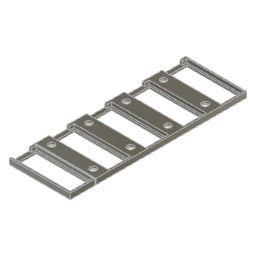
OLED Support for UFC v1 (Autodesk Fusion 360 design; units mm, degrees)
Autodesk Fusion 360 part; units mm, degrees
note: some values were not read from the file. Set by a fixed rule: which face or edge a step refers to.
sketch "Sketch1" plane through (0, 0, 0) normal (0, 0, 1) x (1, 0, 0)
  line L0 (15.1, -5.85) -> (-15.1, -5.85)
  line L1 (-15.1, -5.85) -> (-15.1, 5.85)
  line L2 (-15.1, 5.85) -> (15.1, 5.85)
  line L3 (15.1, 5.85) -> (15.1, -5.85)
  line L4 (15.1, -5.85) -> (-15.1, 5.85) construction
  line L5 (-15.1, -5.85) -> (15.1, 5.85) construction
  line L6 (14.85, -5.4) -> (-14.85, -5.4)
  line L7 (-14.85, -5.4) -> (-14.85, 5.4)
  line L8 (-14.85, 5.4) -> (14.85, 5.4)
  line L9 (14.85, 5.4) -> (14.85, -5.4)
  line L10 (14.85, -5.4) -> (-14.85, 5.4) construction
  line L11 (-14.85, -5.4) -> (14.85, 5.4) construction
  line L12 (16, -7) -> (-16, -7)
  line L13 (-16, -7) -> (-16, 7)
  line L14 (-16, 7) -> (16, 7)
  line L15 (16, 7) -> (16, -7)
  line L16 (16, -7) -> (-16, 7) construction
  line L17 (-16, -7) -> (16, 7) construction
  line L18 (-16, 7) -> (-14.85, 7)
  line L19 (-14.85, 7) -> (-14.85, -3.1641)
  line L20 (-14.85, -3.1641) -> (-16, -3.1641)
  line L21 (-16, -3.1641) -> (-16, 7)
  dimension "d3" = 30.2
  dimension "d4" = 11.7
  dimension "d5" = 29.7
  dimension "d6" = 10.8
  constraint horizontal L0
  constraint perpendicular L0 L1
  constraint parallel L0 L2
  constraint parallel L1 L3
  constraint coincident L4 origin
  constraint coincident L5 origin
  constraint horizontal L6
  constraint perpendicular L6 L7
  constraint parallel L6 L8
  constraint parallel L7 L9
  constraint coincident L10 origin
  constraint coincident L11 origin
  constraint horizontal L12
  constraint perpendicular L12 L13
  constraint parallel L12 L14
  constraint parallel L13 L15
  constraint coincident L16 origin
  constraint coincident L17 origin
  constraint horizontal L18
  constraint vertical L19
  constraint horizontal L20
  constraint vertical L21
  constraint coincident L7 L19.end
  measures "d3" distance of L1.end L2.end
  measures "d4" distance of L0.end L1.end
  measures "d5" distance of L7.end L8.end
  measures "d6" distance of L6.end L7.end
extrude "Extrude1" add sketch "Sketch1" along normal blind 1 contours L0 L1 L2 L3 L6 L7 L8 L9 L19 L20 | L1 L2 L7 L19 L20 makes body 1
extrude "Extrude2" add sketch "Sketch1" along normal blind 4 contours L0 L1 L2 L3 L12 L13 L14 L15 L19 L20 | L1 L2 L13 L14 L18 L19 L20 L21 bodies 1
sketch "Sketch2" plane through (0, 0, 4) normal (0, 0, 1) x (-1, 0, 0)
  line L0 (15.1, -5.85) -> (-15.1, -5.85)
  line L1 (-15.1, -5.85) -> (-15.1, 5.85)
  line L2 (-15.1, 5.85) -> (15.1, 5.85)
  line L3 (15.1, 5.85) -> (15.1, -5.85)
  line L4 (-16, -7) -> (16, -7)
  line L5 (16, -7) -> (16, 7)
  line L6 (16, 7) -> (-16, 7)
  line L7 (-16, 7) -> (-16, -7)
  line L8 (16, 6) -> (15.1, 6)
  line L9 (15.1, 6) -> (15.1, -7)
  line L10 (15.1, -7) -> (16, -7)
  line L11 (16, -7) -> (16, 6)
  constraint horizontal L8
  constraint vertical L9
  constraint horizontal L10
  constraint vertical L11
  constraint coincident L4 L9.end
  constraint coincident L5 L8.start
extrude "Extrude3" cut sketch "Sketch2" against normal blind 4 contours L3 L4 L5 L8 L9 L10 L11 bodies 1
sketch "Sketch3" plane through (-15.1, 0, 0) normal (-1, 0, 0) x (0, -1, 0)
  line L0 (5.85, 1) -> (-5.85, 1)
  line L1 (-5.85, 1) -> (-5.85, 4)
  line L2 (-5.85, 4) -> (-7, 4)
  line L3 (-7, 4) -> (-7, 0)
  line L4 (-7, 0) -> (6, 0)
  line L5 (6, 0) -> (6, 4)
  line L6 (5.85, 4) -> (5.85, 1)
  line L7 (6, 4) -> (5.85, 4)
extrude "Extrude4" add sketch "Sketch3" along normal blind 1 bodies 1
sketch "Sketch4" plane through (0, 5.85, 0) normal (0, -1, 0) x (1, 0, 0)
  line L0 (-16.1, 1) -> (15.1, 1)
  line L1 (15.1, 1) -> (15.1, 4)
  line L2 (15.1, 4) -> (-16.1, 4)
  line L3 (-16.1, 4) -> (-16.1, 1)
  line L4 (-14.8297, 1) -> (-16.1, 1)
  line L5 (-16.1, 1) -> (-16.1, 4)
  line L6 (-16.1, 4) -> (-14.8297, 4)
  line L7 (-14.8297, 4) -> (-14.8297, 1)
  constraint horizontal L4
  constraint vertical L5
  constraint horizontal L6
  constraint vertical L7
  constraint coincident L2.end L3.start
  constraint coincident L0 L4.start
extrude "Extrude5" add sketch "Sketch4" along normal blind 2 contours L0 L2 L3 L4 L5 L6 L7 bodies 1
move_face "OffsetFaces1" offset 1 2 faces at (-16.1, 5.95, 1.6667) (-16, -6.6667, 1.3333) on bodies 1
extrude "Extrude6" cut 1 faces at (-14.8297, 5.0333, 3) along direction (-1, 0, 0) blind 1 on bodies 1 bodies 1
sketch "Sketch5" plane through (0, 0, 0) normal (0, 0, 1) x (1, 0, 0)
  line L0 (15, -6) -> (-15, -6)
  line L1 (-15, -6) -> (-15, 14)
  line L2 (15, 14) -> (15, -6)
  line L3 (15, 54) -> (15, 74)
  line L4 (15, 74) -> (-15, 74)
  line L5 (-15, 74) -> (-15, 54)
  line L6 (-15, -6) -> (15, -6)
  line L7 (15, -6) -> (15, 14.5)
  line L8 (15, 14.5) -> (-15, 14.5)
  line L9 (-15, 14.5) -> (-15, -6)
  line L10 (-15, 14.5) -> (15, 14.5)
  line L11 (15, 14.5) -> (15, 35)
  line L12 (15, 35) -> (-15, 35)
  line L13 (-15, 35) -> (-15, 14.5)
  line L14 (15, 35) -> (15, 55.5)
  line L15 (15, 55.5) -> (-15, 55.5)
  line L16 (-15, 55.5) -> (-15, 35)
  line L17 (-15, 55.5) -> (15, 55.5)
  line L18 (15, 55.5) -> (15, 76)
  line L19 (15, 76) -> (-15, 76)
  line L20 (-15, 76) -> (-15, 55.5)
  dimension "d30" = 30
  dimension "d31" = 20.5
  dimension "d32" = 30
  dimension "d33" = 20.5
  dimension "d34" = 30
  dimension "d35" = 20.5
  dimension "d36" = 30
  dimension "d37" = 20.5
  constraint horizontal L0
  constraint vertical L1
  constraint vertical L2
  constraint vertical L3
  constraint horizontal L4
  constraint vertical L5
  constraint horizontal L6
  constraint vertical L7
  constraint horizontal L8
  constraint vertical L9
  constraint horizontal L10
  constraint vertical L11
  constraint horizontal L12
  constraint vertical L13
  constraint vertical L14
  constraint horizontal L15
  constraint vertical L16
  constraint horizontal L17
  constraint vertical L18
  constraint horizontal L19
  constraint vertical L20
  measures "d30" distance of L0.end L0.start
  measures "d31" distance of L0.end L8.end
  measures "d32" distance of L8.end L7.end
  measures "d33" distance of L8.end L12.end
  measures "d34" distance of L12.end L11.end
  measures "d35" distance of L12.end L15.end
  measures "d36" distance of L15.end L14.end
  measures "d37" distance of L15.end L19.end
copy_body "Body->Comp2" bodies 1 removing the originals makes body 2 in component "Component'"
copy_body "CopyPasteBodies5" bodies 2 makes body 3
move_body "Move5" bodies 3 to x (1, 0, 0) y (0, 1, 0) z (0, 0, 1) at (0, 20.5, 0)
copy_body "CopyPasteBodies6" bodies 3 makes body 4
move_body "Move6" bodies 4 to x (1, 0, 0) y (0, 1, 0) z (0, 0, 1) at (0, 20.5, 0)
copy_body "CopyPasteBodies7" bodies 4 makes body 5
move_body "Move7" bodies 5 to x (1, 0, 0) y (0, 1, 0) z (0, 0, 1) at (0, 20.5, 0)
copy_body "CopyPasteBodies8" bodies 5 makes body 6
move_body "Move8" bodies 6 to x (1, 0, 0) y (0, 1, 0) z (0, 0, 1) at (0, 20.5, 0)
extrude "Extrude12" add 1 faces at (5, 75, 2.6667) along direction (0, -1, 0) blind 7 on bodies 6 bodies 6 5
extrude "Extrude13" add 1 faces at (5, 54.5, 2.6667) along direction (0, -1, 0) blind 8 on bodies 6 bodies 6 4
extrude "Extrude14" add 1 faces at (5, 34, 2.6667) along direction (0, -1, 0) blind 7 on bodies 6 bodies 6 3
extrude "Extrude15" add 1 faces at (5, 13.5, 2.6667) along direction (0, -1, 0) blind 7 on bodies 6 bodies 6
extrude "Extrude16" cut 1 faces at (4.7901, 46.5, 3) along direction (0, 1, 0) blind 0.4 on bodies 6 bodies 6
sketch "Sketch6" plane through (0, 0, 0) normal (0, 0, 1) x (1, 0, 0)
  arc A0 through (-26.4037, -5.2537, 2.667) (-26.7629, -5.1049, 2.667) (-26.9117, -4.7457, 2.667)
  arc A1 through (15.7603, 87.9325, 2.667) (16.1195, 87.7838, 2.667) (16.2683, 87.4245, 2.667)
  circle A2 through (-20.4791, 31.1794, 0.9906) (-22.508, 32.3508, 0.9906) (-22.508, 30.0081, 0.9906)
  arc A3 through (18.3003, -13.0166, 2.667) (18.6595, -12.8678, 2.667) (18.8083, -12.5086, 2.667)
  arc A4 through (-26.4037, 55.7063, 2.667) (-26.7629, 55.8551, 2.667) (-26.9117, 56.2143, 2.667)
  line L0 (13.5696, 95.6954, 0.9906) -> (8.8071, 95.6954, 0.9906)
  line L1 (13.5696, 95.6954, 2.667) -> (18.3003, 95.6954, 2.667)
  arc A5 through (-26.9117, 6.1445, 2.667) (-26.7629, 6.5038, 2.667) (-26.4037, 6.6525, 2.667)
  line L2 (8.8071, 95.6954, 2.667) -> (8.8071, 93.3078, 2.667)
  line L3 (18.8083, 95.1874, 2.667) -> (18.8083, -12.5086, 2.667)
  arc A6 through (8.8071, -10.629, 2.667) (11.1883, -8.2477, 2.667) (13.5696, -10.629, 2.667)
  arc A7 through (15.7603, 67.6125, 2.667) (16.1195, 67.4638, 2.667) (16.2683, 67.1045, 2.667)
  line L4 (-24.2129, -10.629, 2.667) -> (-24.2129, -13.0166, 2.667)
  curve E0
  curve E1
  arc A8 through (-26.9117, 87.4245, 2.667) (-26.7629, 87.7838, 2.667) (-26.4037, 87.9325, 2.667)
  arc A9 through (16.2683, 76.5343, 2.667) (16.1195, 76.1751, 2.667) (15.7603, 76.0263, 2.667)
  circle A10 through (-20.4791, 71.8194, 0.9906) (-22.508, 72.9908, 0.9906) (-22.508, 70.6481, 0.9906)
  arc A11 through (-26.4037, 35.3863, 2.667) (-26.7629, 35.5351, 2.667) (-26.9117, 35.8943, 2.667)
  arc A12 through (-26.9117, 46.7845, 2.667) (-26.7629, 47.1438, 2.667) (-26.4037, 47.2925, 2.667)
  circle A13 through (-20.4791, 93.3078, 0.9906) (-22.508, 94.4792, 0.9906) (-22.508, 92.1365, 0.9906)
  arc A14 through (16.2683, 15.5743, 2.667) (16.1195, 15.2151, 2.667) (15.7603, 15.0663, 2.667)
  line L5 (-26.4037, 76.0263, 2.667) -> (15.7603, 76.0263, 2.667)
  line L6 (-26.4037, 35.3863, 2.667) -> (15.7603, 35.3863, 2.667)
  circle A15 through (12.5409, 51.4994, 0.9906) (10.512, 52.6708, 0.9906) (10.512, 50.3281, 0.9906)
  circle A16 through (8.8071, 10.8594, 2.667) (12.3789, 12.9216, 2.667) (12.3789, 8.7972, 2.667)
  curve E2
  circle A17 through (12.5409, 10.8594, 0.9906) (10.512, 12.0308, 0.9906) (10.512, 9.6881, 0.9906)
  curve E3
  arc A18 through (16.2683, 35.8943, 2.667) (16.1195, 35.5351, 2.667) (15.7603, 35.3863, 2.667)
  line L7 (-24.2129, -13.0166, 2.667) -> (-28.9437, -13.0166, 2.667)
  circle A19 through (12.5409, -10.629, 0.9906) (10.512, -9.4576, 0.9906) (10.512, -11.8003, 0.9906)
  arc A20 through (16.2683, -4.7457, 2.667) (16.1195, -5.1049, 2.667) (15.7603, -5.2537, 2.667)
  arc A21 through (15.7603, 26.9725, 2.667) (16.1195, 26.8238, 2.667) (16.2683, 26.4645, 2.667)
  line L8 (8.8071, -10.629, 2.667) -> (8.8071, -13.0166, 2.667)
  curve E4
  line L9 (13.5696, -13.0166, 2.667) -> (13.5696, -10.629, 2.667)
  arc A22 through (13.5696, 93.3078, 2.667) (11.1883, 90.9266, 2.667) (8.8071, 93.3078, 2.667)
  line L10 (-19.4504, -13.0166, 2.667) -> (-19.4504, -10.629, 2.667)
  arc A23 through (15.7603, 6.6525, 2.667) (16.1195, 6.5038, 2.667) (16.2683, 6.1445, 2.667)
  circle A24 through (12.5409, 71.8194, 0.9906) (10.512, 72.9908, 0.9906) (10.512, 70.6481, 0.9906)
  arc A25 through (-29.4517, -12.5086, 2.667) (-29.3029, -12.8678, 2.667) (-28.9437, -13.0166, 2.667)
  circle A26 through (-24.2129, 10.8594, 2.667) (-20.6411, 12.9216, 2.667) (-20.6411, 8.7972, 2.667)
  circle A27 through (12.5409, 93.3078, 0.9906) (10.512, 94.4792, 0.9906) (10.512, 92.1365, 0.9906)
  arc A28 through (18.8083, 95.1874, 2.667) (18.6595, 95.5466, 2.667) (18.3003, 95.6954, 2.667)
  arc A29 through (-26.9117, 67.1045, 2.667) (-26.7629, 67.4638, 2.667) (-26.4037, 67.6125, 2.667)
  line L11 (13.5696, 93.3078, 2.667) -> (13.5696, 95.6954, 2.667)
  line L12 (-26.4037, 15.0663, 2.667) -> (15.7603, 15.0663, 2.667)
  line L13 (15.7603, 6.6525, 2.667) -> (-26.4037, 6.6525, 2.667)
  circle A30 through (12.5409, 31.1794, 0.9906) (10.512, 32.3508, 0.9906) (10.512, 30.0081, 0.9906)
  line L14 (16.2683, -4.7457, 2.667) -> (16.2683, 6.1445, 2.667)
  line L15 (-29.4517, -12.5086, 2.667) -> (-29.4517, 95.1874, 2.667)
  line L16 (-26.9117, 26.4645, 2.667) -> (-26.9117, 15.5743, 2.667)
  line L17 (-26.4037, -5.2537, 2.667) -> (15.7603, -5.2537, 2.667)
  line L18 (-19.4504, 95.6954, 2.667) -> (8.8071, 95.6954, 2.667)
  line L19 (15.7603, 26.9725, 2.667) -> (-26.4037, 26.9725, 2.667)
  circle A31 through (8.8071, 31.1794, 2.667) (12.3789, 33.2416, 2.667) (12.3789, 29.1172, 2.667)
  circle A32 through (-24.2129, 51.4994, 2.667) (-20.6411, 53.5616, 2.667) (-20.6411, 49.4372, 2.667)
  line L20 (-26.9117, 67.1045, 2.667) -> (-26.9117, 56.2143, 2.667)
  curve E5
  line L21 (16.2683, 15.5743, 2.667) -> (16.2683, 26.4645, 2.667)
  circle A33 through (8.8071, 71.8194, 2.667) (12.3789, 73.8816, 2.667) (12.3789, 69.7572, 2.667)
  circle A34 through (-20.4791, 51.4994, 0.9906) (-22.508, 52.6708, 0.9906) (-22.508, 50.3281, 0.9906)
  arc A35 through (16.2683, 56.2143, 2.667) (16.1195, 55.8551, 2.667) (15.7603, 55.7063, 2.667)
  line L22 (15.7603, 67.6125, 2.667) -> (-26.4037, 67.6125, 2.667)
  line L23 (-26.4037, 55.7063, 2.667) -> (15.7603, 55.7063, 2.667)
  line L24 (8.8071, -13.0166, 0.9906) -> (13.5696, -13.0166, 0.9906)
  line L25 (18.3003, -13.0166, 2.667) -> (13.5696, -13.0166, 2.667)
  arc A36 through (-26.4037, 15.0663, 2.667) (-26.7629, 15.2151, 2.667) (-26.9117, 15.5743, 2.667)
  arc A37 through (-19.4504, 93.3078, 2.667) (-21.8317, 90.9266, 2.667) (-24.2129, 93.3078, 2.667)
  circle A38 through (-20.4791, -10.629, 0.9906) (-22.508, -9.4576, 0.9906) (-22.508, -11.8003, 0.9906)
  circle A39 through (8.8071, 51.4994, 2.667) (12.3789, 53.5616, 2.667) (12.3789, 49.4372, 2.667)
  line L26 (8.8071, -13.0166, 2.667) -> (-19.4504, -13.0166, 2.667)
  arc A40 through (-26.9117, 26.4645, 2.667) (-26.7629, 26.8238, 2.667) (-26.4037, 26.9725, 2.667)
  arc A41 through (15.7603, 47.2925, 2.667) (16.1195, 47.1438, 2.667) (16.2683, 46.7845, 2.667)
  line L27 (16.2683, 76.5343, 2.667) -> (16.2683, 87.4245, 2.667)
  curve E6
  line L28 (-24.2129, 95.6954, 2.667) -> (-24.2129, 93.3078, 2.667)
  line L29 (-26.9117, 46.7845, 2.667) -> (-26.9117, 35.8943, 2.667)
  arc A42 through (-24.2129, -10.629, 2.667) (-21.8317, -8.2477, 2.667) (-19.4504, -10.629, 2.667)
  line L30 (16.2683, 35.8943, 2.667) -> (16.2683, 46.7845, 2.667)
  line L31 (15.7603, 87.9325, 2.667) -> (-26.4037, 87.9325, 2.667)
  line L32 (15.7603, 47.2925, 2.667) -> (-26.4037, 47.2925, 2.667)
  circle A43 through (-24.2129, 71.8194, 2.667) (-20.6411, 73.8816, 2.667) (-20.6411, 69.7572, 2.667)
  line L33 (-26.9117, 6.1445, 2.667) -> (-26.9117, -4.7457, 2.667)
  line L34 (-19.4504, 95.6954, 0.9906) -> (-24.2129, 95.6954, 0.9906)
  line L35 (16.2683, 56.2143, 2.667) -> (16.2683, 67.1045, 2.667)
  arc A44 through (-28.9437, 95.6954, 2.667) (-29.3029, 95.5466, 2.667) (-29.4517, 95.1874, 2.667)
  line L36 (-24.2129, -13.0166, 0.9906) -> (-19.4504, -13.0166, 0.9906)
  circle A45 through (-20.4791, 10.8594, 0.9906) (-22.508, 12.0308, 0.9906) (-22.508, 9.6881, 0.9906)
  line L37 (-28.9437, 95.6954, 2.667) -> (-24.2129, 95.6954, 2.667)
  circle A46 through (-24.2129, 31.1794, 2.667) (-20.6411, 33.2416, 2.667) (-20.6411, 29.1172, 2.667)
  arc A47 through (-26.4037, 76.0263, 2.667) (-26.7629, 76.1751, 2.667) (-26.9117, 76.5343, 2.667)
  curve E7
  line L38 (-26.9117, 87.4245, 2.667) -> (-26.9117, 76.5343, 2.667)
  line L39 (-19.4504, 93.3078, 2.667) -> (-19.4504, 95.6954, 2.667)
sketch "Sketch7" plane through (0, 0, 4) normal (0, 0, 1) x (-1, 0, 0)
  line L0 (15.8297, -44.85) -> (15.8297, -46.9)
  line L1 (15.8297, -46.9) -> (-15.1, -46.9)
  line L2 (-15.1, -46.9) -> (-15.1, -35.15)
  line L3 (-15.1, -35.15) -> (17.1, -35.15)
  line L4 (17.1, -35.15) -> (17.1, -35)
  line L5 (17.1, -35) -> (17, -35)
  line L6 (17, -35) -> (17, -27.5)
  line L7 (17, -27.5) -> (17.1, -27.5)
  line L8 (17.1, -27.5) -> (17.1, -24.35)
  line L9 (17.1, -24.35) -> (15.8297, -24.35)
  line L10 (15.8297, -24.35) -> (15.8297, -26.35)
  line L11 (15.8297, -26.35) -> (-15.1, -26.35)
  line L12 (-15.1, -26.35) -> (-15.1, -14.65)
  line L13 (-15.1, -14.65) -> (17.1, -14.65)
  line L14 (17.1, -14.65) -> (17.1, -14.5)
  line L15 (17.1, -14.5) -> (17, -14.5)
  line L16 (17, -14.5) -> (17, -6.5)
  line L17 (17, -6.5) -> (-16, -6.5)
  line L18 (-16, -6.5) -> (-16, -89)
  line L19 (-16, -89) -> (17.1, -89)
  line L20 (17.1, -89) -> (17.1, -85.85)
  line L21 (17.1, -85.85) -> (15.8297, -85.85)
  line L22 (15.8297, -85.85) -> (15.8297, -87.85)
  line L23 (15.8297, -87.85) -> (-15.1, -87.85)
  line L24 (-15.1, -87.85) -> (-15.1, -76.15)
  line L25 (-15.1, -76.15) -> (17.1, -76.15)
  line L26 (17.1, -76.15) -> (17.1, -76)
  line L27 (17.1, -76) -> (17, -76)
  line L28 (17, -76) -> (17, -68.5)
  line L29 (17, -68.5) -> (17.1, -68.5)
  line L30 (17.1, -68.5) -> (17.1, -65.35)
  line L31 (17.1, -65.35) -> (15.8297, -65.35)
  line L32 (15.8297, -65.35) -> (15.8297, -67.35)
  line L33 (15.8297, -67.35) -> (-15.1, -67.35)
  line L34 (-15.1, -67.35) -> (-15.1, -55.65)
  line L35 (-15.1, -55.65) -> (17.1, -55.65)
  line L36 (17.1, -55.65) -> (17.1, -55.5)
  line L37 (17.1, -55.5) -> (17, -55.5)
  line L38 (17, -55.5) -> (17, -48)
  line L39 (17, -48) -> (17.1, -48)
  line L40 (17.1, -48) -> (17.1, -44.85)
  line L41 (17.1, -44.85) -> (15.8297, -44.85)
  circle A0 through (-8.9129, -71.8194, -1.333) (-11.576, -70.2819, -1.333) (-11.576, -73.3569, -1.333)
  circle A1 through (-8.9383, -51.4994, -1.333) (-11.5633, -49.9839, -1.333) (-11.5633, -53.015, -1.333)
  circle A2 through (-8.9383, -31.1794, -1.333) (-11.5633, -29.6639, -1.333) (-11.5633, -32.695, -1.333)
  circle A3 through (-8.9383, -10.8594, -1.333) (-11.5633, -9.3439, -1.333) (-11.5633, -12.375, -1.333)
  circle A4 centre (12, -71.8138) radius 1.65
  circle A5 centre (12, -51.5037) radius 1.65
  circle A6 centre (12, -31.1822) radius 1.65
  circle A7 centre (12, -10.85) radius 1.65
  dimension "d48" = 3.5
  dimension "d49" = 3.5
  dimension "d50" = 3.5
  dimension "d67" = 3.3
  dimension "d68" = 3.3
  dimension "d69" = 3.3
  dimension "d70" = 3.3
  measures "d67" diameter of A4
  measures "d68" diameter of A5
  measures "d69" diameter of A6
  measures "d70" diameter of A7
extrude "Extrude17" cut sketch "Sketch7" against normal blind 12 contours A3 in plane through (0, 0, 2.667) normal (0, 0, 1) bodies 6
extrude "Extrude18" cut sketch "Sketch7" against normal blind 20 contours A2 in plane through (0, 0, 2.667) normal (0, 0, 1) bodies 6
extrude "Extrude19" cut sketch "Sketch7" against normal blind 13 contours A1 in plane through (0, 0, 2.667) normal (0, 0, 1) bodies 6
extrude "Extrude20" cut sketch "Sketch7" against normal blind 12 contours A0 in plane through (0, 0, 2.667) normal (0, 0, 1) bodies 6
extrude "Extrude21" cut sketch "Sketch7" along normal blind 10 contours A0 in plane through (0, 0, 2.667) normal (0, 0, 1) bodies 6
extrude "Extrude22" cut sketch "Sketch7" along normal blind 10 contours A1 in plane through (0, 0, 2.667) normal (0, 0, 1) bodies 6
extrude "Extrude23" cut sketch "Sketch7" along normal blind 10 contours A2 in plane through (0, 0, 2.667) normal (0, 0, 1) bodies 6
extrude "Extrude24" cut sketch "Sketch7" along normal blind 10 contours A3 in plane through (0, 0, 2.667) normal (0, 0, 1) bodies 6
extrude "Extrude25" cut sketch "Sketch7" against normal blind 10 contours A4 | A5 | A6 | A7 bodies 6
move_face "OffsetFaces1'" offset -2 1 faces at (-5.6432, 6.6167, 4) on bodies 2 in component "Component'"
move_face "OffsetFaces2" offset -2 1 faces at (3.1897, 27.3911, 4) on bodies 6
move_face "OffsetFaces2'" offset -0.5 1 faces at (-5.5198, 5.85, 1.6667) on bodies 2 in component "Component'"
move_face "OffsetFaces3" offset -0.5 4 faces at (4.7901, 87.85, 1.3333) (4.7901, 67.35, 1.3333) (4.7901, 46.9, 1.6667) (4.7901, 26.35, 1.3333) on bodies 6
move_face "OffsetFaces3'" offset -0.2 1 faces at (4.3667, -5.85, 1.6667) on bodies 2 in component "Component'"
move_face "OffsetFaces4" offset -0.2 4 faces at (-6.3667, 76.15, 1.6667) (-6.3667, 55.65, 1.6667) (-6.3667, 35.15, 1.6667) (-6.3667, 14.65, 1.6667) on bodies 6
move_face "OffsetFaces5" offset 1 1 faces at (-15.8833, 10.6, 2) on bodies 6
move_face "OffsetFaces4'" offset 1 1 faces at (-16.6766, 5.7333, 2) on bodies 2 in component "Component'"
chamfer "Chamfer4" distance 2 angle 45 8 edges at (12.3199, 11.4922, 0) (-10.4617, 11.4467, 0) (-10.4617, 31.7788, 0) (-10.4617, 52.1003, 0) (-10.4617, 72.4105, 0) (12.3435, 72.4614, 0) (12.3199, 52.1322, 0) (12.3199, 31.8122, 0) on bodies 6
chamfer "Chamfer1" [suppressed]
copy_body "Body->Comp1" [suppressed] in component "Component"
copy_body "CopyPasteBodies1" [suppressed]
move_body "Move1" [suppressed]
copy_body "CopyPasteBodies2" [suppressed]
move_body "Move2" [suppressed]
copy_body "CopyPasteBodies3" [suppressed]
move_body "Move3" [suppressed]
copy_body "CopyPasteBodies4" [suppressed]
move_body "Move4" [suppressed]
extrude "Extrude7" [suppressed]
extrude "Extrude8" [suppressed]
extrude "Extrude9" [suppressed]
extrude "Extrude10" [suppressed]
extrude "Extrude11" [suppressed]
component "Component'" placed x (1, 0, 0) y (0, 1, 0) z (0, 0, 1) at (0, 0, 0)
